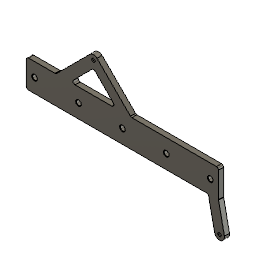
din_mount v4 (Autodesk Fusion 360 design; units mm, degrees)
Autodesk Fusion 360 part; units mm, degrees
sketch "Sketch1" plane through (0, 0, 0) normal (0, 0, 1) x (1, 0, 0)
  line L0 (100, 125) -> (-100, 125)
  line L1 (-100, 125) -> (-100, -125)
  line L2 (-100, -125) -> (100, -125)
  line L3 (100, -125) -> (100, 125)
  line L4 (100, 125) -> (-100, -125) construction
  line L5 (-100, 125) -> (100, -125) construction
  line L6 (-100, 125) -> (100, 125)
  line L7 (100, 125) -> (100, 129)
  line L8 (100, 129) -> (-100, 129)
  line L9 (-100, 129) -> (-100, 125)
  line L10 (-100, -125) -> (100, -125)
  line L11 (100, -125) -> (100, -129)
  line L12 (100, -129) -> (-100, -129)
  line L13 (-100, -129) -> (-100, -125)
  line L14 (100, 125) -> (104, 125)
  line L15 (104, 125) -> (104, -125)
  line L16 (104, -125) -> (100, -125)
  line L17 (100, -125) -> (100, 125)
  line L18 (-100, 125) -> (-104, 125)
  line L19 (-104, 125) -> (-104, -125)
  line L20 (-104, -125) -> (-100, -125)
  line L21 (-100, -125) -> (-100, 125)
  line L22 (-80, -53.8) -> (-80, 2.2) construction
  circle A0 centre (-80, -53.8) radius 1.65 construction
  circle A1 centre (-80, 2.2) radius 1.65 construction
  line L23 (-61.0622, -1) -> (-98.9378, -1) construction
  line L24 (-98.9378, -1) -> (-98.9378, -50.6) construction
  line L25 (-98.9378, -50.6) -> (-61.0622, -50.6) construction
  line L26 (-61.0622, -50.6) -> (-61.0622, -1) construction
  line L27 (-61.0622, -1) -> (-98.9378, -50.6) construction
  line L28 (-98.9378, -1) -> (-61.0622, -50.6) construction
  line L29 (-30.5, 49.5) -> (98.5, 49.5) construction
  line L30 (98.5, 49.5) -> (98.5, -47.5) construction
  line L31 (98.5, -47.5) -> (-30.5, -47.5) construction
  line L32 (-30.5, -47.5) -> (-30.5, 49.5) construction
  circle A2 centre (-28, 43) radius 1.65
  circle A3 centre (94, -42) radius 1.65
  line L33 (-100, 125) -> (-85.5, 125)
  line L34 (-85.5, 125) -> (-85.5, 116)
  line L35 (-85.5, 116) -> (-100, 116)
  line L36 (-100, 116) -> (-100, 125)
  line L37 (100, 125) -> (85.5, 125)
  line L38 (85.5, 125) -> (85.5, 116)
  line L39 (85.5, 116) -> (100, 116)
  line L40 (100, 116) -> (100, 125)
  line L41 (-100, -125) -> (-85.5, -125)
  line L42 (-85.5, -125) -> (-85.5, -116)
  line L43 (-85.5, -116) -> (-100, -116)
  line L44 (-100, -116) -> (-100, -125)
  line L45 (100, -125) -> (85.5, -125)
  line L46 (85.5, -125) -> (85.5, -116)
  line L47 (85.5, -116) -> (100, -116)
  line L48 (100, -116) -> (100, -125)
  line L49 (-100, 100) -> (-104, 100)
  line L50 (100, 100) -> (104, 100)
  line L51 (-100, -100) -> (-104, -100)
  line L52 (100, -100) -> (104, -100)
  line L53 (-85.5, 125) -> (-85.5, 129)
  line L54 (85.5, 125) -> (85.5, 129)
  line L55 (-85.5, -125) -> (-85.5, -129)
  line L56 (85.5, -125) -> (85.5, -129)
  line L57 (-115, -140) -> (-75, -140) construction
  line L58 (-75, -140) -> (-75, -87) construction
  line L59 (-75, -87) -> (-115, -87) construction
  line L60 (-115, -87) -> (-115, -140) construction
  line L61 (-63.3606, -140) -> (-21.3606, -140) construction
  line L62 (-21.3606, -140) -> (-21.3606, -53.8) construction
  line L63 (-21.3606, -53.8) -> (-63.3606, -53.8) construction
  line L64 (-63.3606, -53.8) -> (-63.3606, -140) construction
  line L65 (-100, 0) -> (-118.2487, 0) construction
  circle A4 centre (0, 0) radius 152.5
  circle A5 centre (-85, -72) radius 1.65
  line L66 (-85, -72) -> (85, -72) construction
  line L67 (85, -72) -> (85, 72) construction
  line L68 (85, 72) -> (-85, 72) construction
  line L69 (-85, 72) -> (-85, -72) construction
  circle A6 centre (85, 72) radius 1.65
  circle A7 centre (85, -72) radius 1.65
  circle A8 centre (-85, 72) radius 1.65
  point P0 (-80, -25.8)
  dimension "d1" = 200
  dimension "d2" = 250
  dimension "d3" = 4
  dimension "d4" = 4
  dimension "d5" = 4
  dimension "d6" = 4
  dimension "d7" = 20
  dimension "d8" = 56
  dimension "d10" = 3.3
  dimension "d11" = 37.8755
  dimension "d12" = 49.6
  dimension "d13" = 2.5
  dimension "d14" = 6.5
  dimension "d15" = 3.3
  dimension "d16" = 5.5
  dimension "d17" = 4.5
  dimension "d18" = 129
  dimension "d19" = 97
  dimension "d20" = 1.5
  dimension "d21" = 14.5
  dimension "d22" = 9
  dimension "d23" = 14.5
  dimension "d24" = 9
  dimension "d25" = 14.5
  dimension "d26" = 14.5
  dimension "d27" = 9
  dimension "d28" = 9
  dimension "d29" = 25
  dimension "d30" = 25
  dimension "d31" = 25
  dimension "d32" = 25
  dimension "d33" = 40
  dimension "d34" = 53
  dimension "d35" = 15
  dimension "d36" = 15
  dimension "d37" = 3.3
  dimension "d38" = 86.2
  dimension "d39" = 42
  dimension "d40" = 1
  dimension "d50" = 305
  dimension "d51" = 3.3
  dimension "d52" = 15
  dimension "d53" = 15
  dimension "d54" = 15
  dimension "d55" = 53
  dimension "d56" = 53
  dimension "d57" = 170
  dimension "d58" = 144
  dimension "d60" = 47.5
  dimension "d61" = 49.5
  constraint horizontal L0
  constraint perpendicular L0 L1
  constraint parallel L0 L2
  constraint parallel L1 L3
  constraint coincident L4 A4.centre
  constraint coincident L5 A4.centre
  constraint coincident A4.centre origin
  constraint horizontal L6
  constraint vertical L7
  constraint horizontal L8
  constraint vertical L9
  constraint horizontal L10
  constraint vertical L11
  constraint horizontal L12
  constraint vertical L13
  constraint horizontal L14
  constraint vertical L15
  constraint horizontal L16
  constraint vertical L17
  constraint horizontal L18
  constraint vertical L19
  constraint horizontal L20
  constraint vertical L21
  constraint coincident L22.start A0.centre
  constraint coincident L22.end A1.centre
  constraint equal A0 A1
  constraint horizontal L23
  constraint perpendicular L23 L24
  constraint parallel L23 L25
  constraint parallel L24 L26
  constraint coincident L27 P0
  constraint coincident L28 P0
  constraint midpoint L22 P0
  constraint collinear L2 L20
  constraint collinear L11 L17
  constraint collinear L7 L17
  constraint horizontal L29
  constraint vertical L30
  constraint horizontal L31
  constraint vertical L32
  constraint equal A2 A3
  constraint horizontal L33
  constraint vertical L34
  constraint horizontal L35
  constraint vertical L36
  constraint horizontal L37
  constraint vertical L38
  constraint horizontal L39
  constraint vertical L40
  constraint horizontal L41
  constraint vertical L42
  constraint horizontal L43
  constraint vertical L44
  constraint horizontal L45
  constraint vertical L46
  constraint horizontal L47
  constraint vertical L48
  constraint coincident L1 L49.start
  constraint coincident L19 L49.end
  constraint perpendicular L19 L49
  constraint coincident L3 L50.start
  constraint coincident L15 L50.end
  constraint perpendicular L15 L50
  constraint coincident L21 L51.start
  constraint coincident L19 L51.end
  constraint perpendicular L19 L51
  constraint coincident L17 L52.start
  constraint coincident L15 L52.end
  constraint perpendicular L15 L52
  constraint coincident L8 L53.end
  constraint perpendicular L8 L53
  constraint coincident L8 L54.end
  constraint perpendicular L8 L54
  constraint coincident L12 L55.end
  constraint perpendicular L12 L55
  constraint coincident L12 L56.end
  constraint perpendicular L12 L56
  constraint horizontal L57
  constraint vertical L58
  constraint horizontal L59
  constraint vertical L60
  constraint horizontal L61
  constraint vertical L62
  constraint horizontal L63
  constraint vertical L64
  constraint vertical L22
  constraint midpoint L21 L65.start
  constraint perpendicular L19 L65
  constraint collinear L57 L61
  constraint horizontal L66
  constraint vertical L67
  constraint horizontal L68
  constraint vertical L69
  constraint coincident A5.centre L66.start
  constraint coincident L67.end L68.start
  constraint coincident L66.end L67.start
  constraint coincident L68.end L69.start
  constraint equal A6 A8
  constraint equal A5 A7
  constraint equal A6 A7
  measures "d1" distance of L0.start L0.end
  measures "d2" distance of L0.start L2.end
  measures "d3" distance of L0 L8
  measures "d4" distance of L2.end L11.end
  measures "d5" distance of L0.start L14.end
  measures "d6" distance of L0.end L18.end
  measures "d7" distance of L1 L22.start
  measures "d8" distance of L22.start L22.end
  measures "d10" diameter of A1
  measures "d11" distance of L23.start L23.end
  measures "d12" distance of L23.start L25.end
  measures "d13" distance of L32 A2.centre
  measures "d14" distance of L29 A2.centre
  measures "d15" diameter of A2
  measures "d16" distance of L31 A3.centre
  measures "d17" distance of L30 A3.centre
  measures "d18" distance of L29.start L29.end
  measures "d19" distance of L29.end L30.end
  measures "d20" distance of L17 L30
  measures "d21" distance of L34.end L35.end
  measures "d22" distance of L33.end L34.end
  measures "d23" distance of L38.end L39.end
  measures "d24" distance of L37.end L38.end
  measures "d25" distance of L42.end L43.end
  measures "d26" distance of L46.end L47.end
  measures "d27" distance of L41.end L42.end
  measures "d28" distance of L45.end L46.end
  measures "d29" distance of L20 L51
  measures "d30" distance of L18 L49
  measures "d31" distance of L14 L50
  measures "d32" distance of L10 L52
  measures "d33" distance of L57.start L57.end
  measures "d34" distance of L57.start L59.end
  measures "d35" distance of L10 L57
  measures "d36" distance of L21 L60
  measures "d37" diameter of A3
  measures "d38" distance of L61.end L62.end
  measures "d39" distance of L61.start L61.end
  measures "d40" distance of L23 L65
  measures "d50" diameter of A4
  measures "d51" diameter of A5
  measures "d52" distance of L1 A5.centre
  measures "d53" distance of L59 A5.centre
  measures "d54" distance of L17 L67
  measures "d55" distance of L10 L66
  measures "d56" distance of L6 L68
  measures "d57" distance of L67.end L68.end
  measures "d58" distance of L66.end L67.end
  measures "d60" distance of L31 L65
  measures "d61" distance of L29 L65
extrude "Extrude1" add sketch "Sketch1" along normal blind 3 contours L0 L1 L2 L3 L6 L10 L17 L21 L34 L35 L38 L39 L42 L43 L46 L47 A4 | L0 L6 L8 L53 L54 A4 | L3 L15 L17 L50 L52 | L1 L19 L21 L49 L51 | L2 L10 L12 L55 L56 A4 makes body 1
sketch "Sketch2" plane through (0, 0, 3) normal (0, 0, 1) x (1, 0, 0)
  circle A0 centre (85, -72) radius 1.65
  circle A1 centre (-85, -72) radius 1.65
  circle A2 centre (85, 72) radius 1.65
  circle A3 centre (94, -42) radius 1.65
  circle A4 centre (-85, 72) radius 1.65
  circle A5 centre (-28, 43) radius 1.65
  line L0 (100, 100) -> (100, 115.1358)
  arc A6 (100, 115.1358) -> (98.9962, 116) centre (0, 0) ccw
  line L1 (98.9962, 116) -> (85.5, 116)
  line L2 (85.5, 116) -> (85.5, 126.2775)
  arc A7 (85.5, 126.2775) -> (81.3342, 129) centre (0, 0) ccw
  line L3 (81.3342, 129) -> (-81.3342, 129)
  arc A8 (-81.3342, 129) -> (-85.5, 126.2775) centre (0, 0) ccw
  line L4 (-85.5, 126.2775) -> (-85.5, 116)
  line L5 (-85.5, 116) -> (-98.9962, 116)
  arc A9 (-98.9962, 116) -> (-100, 115.1358) centre (0, 0) ccw
  line L6 (-100, 115.1358) -> (-100, 100)
  line L7 (-100, 100) -> (-104, 100)
  line L8 (-104, 100) -> (-104, -100)
  line L9 (-104, -100) -> (-100, -100)
  line L10 (-100, -100) -> (-100, -115.1358)
  arc A10 (-100, -115.1358) -> (-98.9962, -116) centre (0, 0) ccw
  line L11 (-98.9962, -116) -> (-85.5, -116)
  line L12 (-85.5, -116) -> (-85.5, -126.2775)
  arc A11 (-85.5, -126.2775) -> (-81.3342, -129) centre (0, 0) ccw
  line L13 (-81.3342, -129) -> (81.3342, -129)
  arc A12 (81.3342, -129) -> (85.5, -126.2775) centre (0, 0) ccw
  line L14 (85.5, -126.2775) -> (85.5, -116)
  line L15 (85.5, -116) -> (98.9962, -116)
  arc A13 (98.9962, -116) -> (100, -115.1358) centre (0, 0) ccw
  line L16 (100, -115.1358) -> (100, -100)
  line L17 (100, -100) -> (104, -100)
  line L18 (104, -100) -> (104, 100)
  line L19 (104, 100) -> (100, 100)
  line L20 (-10, 129) -> (10, 129)
  line L21 (10, 129) -> (10, 111)
  line L22 (8, 109) -> (-8, 109)
  line L23 (-10, 111) -> (-10, 129)
  arc A14 (-10, 111) -> (-8, 109) centre (-8, 111) ccw
  arc A15 (8, 109) -> (10, 111) centre (8, 111) ccw
  point P0 (10, 109)
  point P1 (-10, 109)
  dimension "d62" = 20
  dimension "d63" = 20
  dimension "d64" = 2
  constraint horizontal L20
  constraint vertical L21
  constraint horizontal L22
  constraint vertical L23
  constraint coincident L3 L20.start
  constraint midpoint L3 L20
  constraint coincident P1 L22
  constraint coincident P1 L23
  constraint tangent L22 A14
  constraint tangent L23 A14
  constraint coincident P0 L21
  constraint coincident P0 L22
  constraint tangent L21 A15
  constraint tangent L22 A15
  constraint equal A14 A15
  measures "d62" distance of L20.start P1
  measures "d63" distance of P0 P1
  measures "d64" radius of A14
extrude "Extrude2" cut sketch "Sketch2" against normal blind 3 contours L3 L20 L21 L22 L23 A14 A15 bodies 1
fillet "Fillet4" radius 2 2 edges at (-10, 129, 1.5) (10, 129, 1.5) on bodies 1
sketch "Sketch3" plane through (0, 0, 3) normal (0, 0, 1) x (1, 0, 0)
  arc A0 (12, 129) -> (10, 127) centre (12, 127) ccw
  line L0 (10, 127) -> (10, 111)
  arc A1 (8, 109) -> (10, 111) centre (8, 111) ccw
  line L1 (8, 109) -> (-8, 109)
  arc A2 (-10, 111) -> (-8, 109) centre (-8, 111) ccw
  line L2 (-10, 111) -> (-10, 127)
  arc A3 (-10, 127) -> (-12, 129) centre (-12, 127) ccw
  line L3 (-12, 129) -> (-81.3342, 129)
  arc A4 (-81.3342, 129) -> (-85.5, 126.2775) centre (0, 0) ccw
  line L4 (-85.5, 126.2775) -> (-85.5, 116)
  line L5 (-85.5, 116) -> (-98.9962, 116)
  arc A5 (-98.9962, 116) -> (-100, 115.1358) centre (0, 0) ccw
  line L6 (-100, 115.1358) -> (-100, 100)
  line L7 (-100, 100) -> (-104, 100)
  line L8 (-104, 100) -> (-104, -100)
  line L9 (-104, -100) -> (-100, -100)
  line L10 (-100, -100) -> (-100, -115.1358)
  arc A6 (-100, -115.1358) -> (-98.9962, -116) centre (0, 0) ccw
  line L11 (-98.9962, -116) -> (-85.5, -116)
  line L12 (-85.5, -116) -> (-85.5, -126.2775)
  arc A7 (-85.5, -126.2775) -> (-81.3342, -129) centre (0, 0) ccw
  line L13 (-81.3342, -129) -> (81.3342, -129)
  arc A8 (81.3342, -129) -> (85.5, -126.2775) centre (0, 0) ccw
  line L14 (85.5, -126.2775) -> (85.5, -116)
  line L15 (85.5, -116) -> (98.9962, -116)
  arc A9 (98.9962, -116) -> (100, -115.1358) centre (0, 0) ccw
  line L16 (100, -115.1358) -> (100, -100)
  line L17 (100, -100) -> (104, -100)
  line L18 (104, -100) -> (104, 100)
  line L19 (104, 100) -> (100, 100)
  line L20 (100, 100) -> (100, 115.1358)
  arc A10 (100, 115.1358) -> (98.9962, 116) centre (0, 0) ccw
  line L21 (98.9962, 116) -> (85.5, 116)
  line L22 (85.5, 116) -> (85.5, 126.2775)
  arc A11 (85.5, 126.2775) -> (81.3342, 129) centre (0, 0) ccw
  line L23 (81.3342, 129) -> (12, 129)
  circle A12 centre (85, -72) radius 1.65
  circle A13 centre (-85, -72) radius 1.65
  circle A14 centre (85, 72) radius 1.65
  circle A15 centre (94, -42) radius 1.65
  circle A16 centre (-85, 72) radius 1.65
  circle A17 centre (-28, 43) radius 1.65
  circle A18 centre (0, 59) radius 6
  dimension "d69" = 12
  dimension "d70" = 50
  dimension "d71" = 104
  measures "d69" diameter of A18
  measures "d70" distance of L1 A18.centre
  measures "d71" distance of L8 A18.centre
extrude "Extrude3" cut sketch "Sketch3" against normal blind 3 contours A18 bodies 1
sketch "Sketch4" plane through (0, 0, 3) normal (0, 0, 1) x (1, 0, 0)
  circle A0 centre (0, 59) radius 6
  arc A1 (12, 129) -> (10, 127) centre (12, 127) ccw
  line L0 (10, 127) -> (10, 111)
  arc A2 (8, 109) -> (10, 111) centre (8, 111) ccw
  line L1 (8, 109) -> (-8, 109)
  arc A3 (-10, 111) -> (-8, 109) centre (-8, 111) ccw
  line L2 (-10, 111) -> (-10, 127)
  arc A4 (-10, 127) -> (-12, 129) centre (-12, 127) ccw
  line L3 (-12, 129) -> (-81.3342, 129)
  arc A5 (-81.3342, 129) -> (-85.5, 126.2775) centre (0, 0) ccw
  line L4 (-85.5, 126.2775) -> (-85.5, 116)
  line L5 (-85.5, 116) -> (-98.9962, 116)
  arc A6 (-98.9962, 116) -> (-100, 115.1358) centre (0, 0) ccw
  line L6 (-100, 115.1358) -> (-100, 100)
  line L7 (-100, 100) -> (-104, 100)
  line L8 (-104, 100) -> (-104, -100)
  line L9 (-104, -100) -> (-100, -100)
  line L10 (-100, -100) -> (-100, -115.1358)
  arc A7 (-100, -115.1358) -> (-98.9962, -116) centre (0, 0) ccw
  line L11 (-98.9962, -116) -> (-85.5, -116)
  line L12 (-85.5, -116) -> (-85.5, -126.2775)
  arc A8 (-85.5, -126.2775) -> (-81.3342, -129) centre (0, 0) ccw
  line L13 (-81.3342, -129) -> (81.3342, -129)
  arc A9 (81.3342, -129) -> (85.5, -126.2775) centre (0, 0) ccw
  line L14 (85.5, -126.2775) -> (85.5, -116)
  line L15 (85.5, -116) -> (98.9962, -116)
  arc A10 (98.9962, -116) -> (100, -115.1358) centre (0, 0) ccw
  line L16 (100, -115.1358) -> (100, -100)
  line L17 (100, -100) -> (104, -100)
  line L18 (104, -100) -> (104, 100)
  line L19 (104, 100) -> (100, 100)
  line L20 (100, 100) -> (100, 115.1358)
  arc A11 (100, 115.1358) -> (98.9962, 116) centre (0, 0) ccw
  line L21 (98.9962, 116) -> (85.5, 116)
  line L22 (85.5, 116) -> (85.5, 126.2775)
  arc A12 (85.5, 126.2775) -> (81.3342, 129) centre (0, 0) ccw
  line L23 (81.3342, 129) -> (12, 129)
  circle A13 centre (85, -72) radius 1.65
  circle A14 centre (-85, -72) radius 1.65
  circle A15 centre (85, 72) radius 1.65
  circle A16 centre (94, -42) radius 1.65
  circle A17 centre (-85, 72) radius 1.65
  circle A18 centre (-28, 43) radius 1.65
sketch "Sketch5" plane through (0, 0, 3) normal (0, 0, 1) x (1, 0, 0)
  circle A0 centre (0, 59) radius 6
  arc A1 (12, 129) -> (10, 127) centre (12, 127) ccw
  line L0 (10, 127) -> (10, 111)
  arc A2 (8, 109) -> (10, 111) centre (8, 111) ccw
  line L1 (8, 109) -> (-8, 109)
  arc A3 (-10, 111) -> (-8, 109) centre (-8, 111) ccw
  line L2 (-10, 111) -> (-10, 127)
  arc A4 (-10, 127) -> (-12, 129) centre (-12, 127) ccw
  line L3 (-12, 129) -> (-81.3342, 129)
  arc A5 (-81.3342, 129) -> (-85.5, 126.2775) centre (0, 0) ccw
  line L4 (-85.5, 126.2775) -> (-85.5, 116)
  line L5 (-85.5, 116) -> (-98.9962, 116)
  arc A6 (-98.9962, 116) -> (-100, 115.1358) centre (0, 0) ccw
  line L6 (-100, 115.1358) -> (-100, 100)
  line L7 (-100, 100) -> (-104, 100)
  line L8 (-104, 100) -> (-104, -100)
  line L9 (-104, -100) -> (-100, -100)
  line L10 (-100, -100) -> (-100, -115.1358)
  arc A7 (-100, -115.1358) -> (-98.9962, -116) centre (0, 0) ccw
  line L11 (-98.9962, -116) -> (-85.5, -116)
  line L12 (-85.5, -116) -> (-85.5, -126.2775)
  arc A8 (-85.5, -126.2775) -> (-81.3342, -129) centre (0, 0) ccw
  line L13 (-81.3342, -129) -> (81.3342, -129)
  arc A9 (81.3342, -129) -> (85.5, -126.2775) centre (0, 0) ccw
  line L14 (85.5, -126.2775) -> (85.5, -116)
  line L15 (85.5, -116) -> (98.9962, -116)
  arc A10 (98.9962, -116) -> (100, -115.1358) centre (0, 0) ccw
  line L16 (100, -115.1358) -> (100, -100)
  line L17 (100, -100) -> (104, -100)
  line L18 (104, -100) -> (104, 100)
  line L19 (104, 100) -> (100, 100)
  line L20 (100, 100) -> (100, 115.1358)
  arc A11 (100, 115.1358) -> (98.9962, 116) centre (0, 0) ccw
  line L21 (98.9962, 116) -> (85.5, 116)
  line L22 (85.5, 116) -> (85.5, 126.2775)
  arc A12 (85.5, 126.2775) -> (81.3342, 129) centre (0, 0) ccw
  line L23 (81.3342, 129) -> (12, 129)
  circle A13 centre (85, -72) radius 1.65
  circle A14 centre (-85, -72) radius 1.65
  circle A15 centre (85, 72) radius 1.65
  circle A16 centre (94, -42) radius 1.65
  circle A17 centre (-85, 72) radius 1.65
  circle A18 centre (-28, 43) radius 1.65
  circle A19 centre (94, -42) radius 2.35
  circle A20 centre (-28, 43) radius 1.65
  circle A21 centre (-28, 43) radius 2.35
  circle A22 centre (94, -42) radius 1.65
  circle A23 centre (94, -42) radius 4.85
  circle A24 centre (-28, 43) radius 4.85
  circle A25 centre (0, 0) radius 1.65
  circle A26 centre (0, 0) radius 2.35
  circle A27 centre (-85, 0) radius 2.35
  circle A28 centre (-85, 0) radius 1.65
  circle A29 centre (-42.5, 0) radius 2.35
  circle A30 centre (-42.5, 0) radius 1.65
  circle A31 centre (42.5, 0) radius 2.35
  circle A32 centre (42.5, 0) radius 1.65
  circle A33 centre (85, 0) radius 2.35
  circle A34 centre (85, 0) radius 1.65
  line L24 (81.4652, -13.5) -> (-91, -13.5)
  line L25 (-93, -11.5) -> (-93, 11.5)
  line L26 (-91, 13.5) -> (-65.1874, 13.5)
  line L27 (93, 11.5) -> (93, -13.2933)
  line L28 (93.0423, -13.7023) -> (98.7475, -41.0081)
  line L29 (89.2525, -42.9919) -> (83.4229, -15.091)
  line L30 (7.7731, 14.0858) -> (-24.5705, 46.4295)
  line L31 (8.3589, 13.5) -> (-10.1874, 13.5) construction
  line L32 (-26.5858, 34.7269) -> (-8.7731, 16.9142)
  line L33 (-63.7731, 14.0858) -> (-31.4295, 46.4295)
  line L34 (-64.3589, 13.5) -> (-45.8126, 13.5) construction
  line L35 (-47.2269, 16.9142) -> (-29.4142, 34.7269)
  arc A35 (83.4229, -15.091) -> (81.4652, -13.5) centre (81.4652, -15.5) ccw
  arc A36 (93, -13.2933) -> (93.0423, -13.7023) centre (95, -13.2933) ccw
  arc A37 (93, 11.5) -> (91, 13.5) centre (91, 11.5) ccw
  arc A38 (-93, -11.5) -> (-91, -13.5) centre (-91, -11.5) ccw
  arc A39 (-91, 13.5) -> (-93, 11.5) centre (-91, 11.5) ccw
  arc A40 (-65.1874, 13.5) -> (-63.7731, 14.0858) centre (-65.1874, 15.5) ccw
  arc A41 (-47.2269, 16.9142) -> (-45.8126, 13.5) centre (-45.8126, 15.5) ccw
  arc A42 (-26.5858, 34.7269) -> (-29.4142, 34.7269) centre (-28, 33.3126) ccw
  arc A43 (-10.1874, 13.5) -> (-8.7731, 16.9142) centre (-10.1874, 15.5) ccw
  line L36 (91, 13.5) -> (9.1874, 13.5)
  arc A44 (7.7731, 14.0858) -> (9.1874, 13.5) centre (9.1874, 15.5) ccw
  line L37 (-10.1874, 13.5) -> (-45.8126, 13.5)
  line L38 (-45.8126, 13.5) -> (-10.1874, 13.5) construction
  point P0 (-85, 0)
  point P1 (-85, 0)
  point P2 (-42.5, 0)
  point P3 (-42.5, 0)
  point P4 (42.5, 0)
  point P5 (42.5, 0)
  point P6 (85, 0)
  point P7 (85, 0)
  dimension "d74" = 4.7
  dimension "d75" = 3.3
  dimension "d76" = 4.7
  dimension "d80" = 3.3
  dimension "d81" = 9.7
  dimension "d82" = 9.7
  dimension "d83" = 3.3
  dimension "d84" = 4.7
  dimension "d87" = 85
  dimension "d88" = 85
  dimension "d89" = 8
  dimension "d90" = 8
  dimension "d91" = 13.5
  dimension "d92" = 13.5
  dimension "d93" = 45
  dimension "d94" = 45
  dimension "d95" = 2
  dimension "d96" = 2
  dimension "d98" = 2
  dimension "d99" = 2
  dimension "d100" = 2
  dimension "d101" = 2
  dimension "d102" = 2
  dimension "d103" = 2
  dimension "d104" = 2
  constraint concentric A18 A20
  constraint concentric A20 A21
  constraint concentric A19 A22
  constraint concentric A20 A24
  constraint concentric A5 A25
  constraint concentric A25 A26
  constraint horizontal L24
  constraint vertical L25
  constraint horizontal L26
  constraint vertical L27
  constraint coincident A23 L28.end
  constraint tangent A23 L28
  constraint coincident A23 L29.start
  constraint tangent A23 L29
  constraint parallel L28 L29
  constraint horizontal L31
  constraint coincident L26 L31.start
  constraint tangent A24 L30
  constraint coincident A24 L30.end
  constraint parallel L30 L32
  constraint tangent A24 L32
  constraint horizontal L34
  constraint coincident L26 L34.start
  constraint perpendicular L30 L35
  constraint tangent A24 L33
  constraint coincident A24 L33.end
  constraint tangent A24 L35
  constraint tangent L29 A35
  constraint tangent L24 A35
  constraint tangent L27 A36
  constraint tangent L28 A36
  constraint tangent L26 A37
  constraint tangent L27 A37
  constraint tangent L24 A38
  constraint tangent L25 A38
  constraint tangent L25 A39
  constraint tangent L26 A39
  constraint equal A38 A39
  constraint coincident L34.start L33
  constraint coincident L26 A37.end
  constraint tangent L33 A40
  constraint tangent L26 A40
  constraint tangent L35 A41
  constraint tangent L31 A41
  constraint tangent L35 A42
  constraint tangent L32 A42
  constraint tangent L32 A43
  constraint tangent L34 A43
  constraint coincident L31.start L36
  constraint coincident L31.start L30
  constraint tangent L36 A44
  constraint tangent L30 A44
  constraint horizontal L38
  measures "d74" diameter of A19
  measures "d75" diameter of A20
  measures "d76" diameter of A21
  measures "d80" diameter of A22
  measures "d81" diameter of A23
  measures "d82" diameter of A24
  measures "d83" diameter of A25
  measures "d84" diameter of A26
  measures "d89" distance of P7 L27
  measures "d90" distance of P1 L25
  measures "d91" distance of P1 L24
  measures "d92" distance of P1 L26
  measures "d93" angle of L30 L31
  measures "d94" angle of L33 L34
  measures "d95" radius of A35
  measures "d96" radius of A36
  measures "d98" radius of A37
  measures "d99" radius of A38
  measures "d100" radius of A40
  measures "d101" radius of A41
  measures "d102" radius of A42
  measures "d103" radius of A43
  measures "d104" radius of A44
extrude "Extrude4" add sketch "Sketch5" along normal blind 5 separate body contours A23 | A23 A24 L24 L25 L26 L27 L28 L29 L30 L33 A35 A36 A37 A38 A39 A40 L36 A44 | A24 makes body 2
extrude "Extrude5" add sketch "Sketch5" along normal blind 5 contours A19 | A21 bodies 2
extrude "Extrude6" cut sketch "Sketch5" along normal blind 4 contours A19 | A21 bodies 2
chamfer "Chamfer2" distance 0.4 angle 45 2 edges at (91.809, -42.8498, 3) (-30.191, 42.1502, 3) on bodies 2
extrude "Extrude7" add sketch "Sketch5" along normal blind 1 contours A26 | A27 | A29 | A31 | A33 bodies 2
chamfer "Chamfer3" distance 0.4 angle 45 5 edges at (82.809, 0.8498, 8) (40.309, 0.8498, 8) (-2.191, 0.8498, 8) (-44.691, 0.8498, 8) (-87.191, 0.8498, 8) on bodies 2
hidden bodies 1
equation "d4 = d3"
equation "d5 = d3"
equation "d6 = d3"
equation "d23 = d21"
equation "d24 = d22"
equation "d25 = d21"
equation "d26 = d25"
equation "d27 = d22"
equation "d28 = d24"
equation "d30 = d29"
equation "d31 = d29"
equation "d32 = d29"
equation "d36 = d35"
equation "d60 = d19 / 2 - 1 mm"
equation "d74 = outer_heat"
equation "d75 = inner_heat"
equation "d76 = outer_heat"
equation "inner_heat = 3.3 mm"
equation "outer_heat = 4.7 mm"
equation "cir_offset = 5 mm"
equation "d80 = inner_heat"
equation "d81 = outer_heat + cir_offset"
equation "d82 = outer_heat + cir_offset"
equation "d83 = inner_heat"
equation "d84 = outer_heat"
equation "d91 = ( 27 / 2 ) * 1 mm"
equation "d92 = ( 27 / 2 ) * 1 mm"
equation "d95 = fillet"
equation "d96 = fillet"
equation "fillet = 2 mm"
equation "d98 = fillet"
equation "d99 = fillet"
equation "d100 = fillet"
equation "d101 = fillet"
equation "d102 = fillet"
equation "d103 = fillet"
equation "d104 = fillet"
